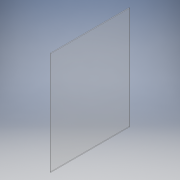
# Autodesk Inventor part: PanelThree
Saved by Autodesk Inventor 2017 (Build 210142000, 142)
## iProperties
Created: 2020-02-22
Part Number: PanelThree
Material: Polycarbonate, Clear
Document SubType Name: Modeling
Designer: S338674153
Density: 1.2 g/cm^3
Appearance: Polycarbonate - Clear
Author: S338674153
Autodesk Inventor part; units mm, degrees
ref_plane "YZ Plane" through (0, 0, 0) normal (1, 0, 0) x (0, 1, 0)
ref_plane "XZ Plane" through (0, 0, 0) normal (0, 1, 0) x (-1, 0, 0)
ref_plane "XY Plane" through (0, 0, 0) normal (0, 0, 1) x (1, 0, 0)
sketch "Sketch1" plane through (0, 0, 0) normal (0, 1, 0) x (-1, 0, 0)
  line L0 (0, 0) -> (2.54, 0)
  line L1 (2.54, 0) -> (2.54, -254)
  line L2 (2.54, -254) -> (0, -254)
  line L3 (0, -254) -> (0, 0)
  dimension "d0" = 254
  dimension "d1" = 2.54
  constraints: 8 end point, 2 parallel, 1 horizontal, 1 perpendicular
  measures "d0" distance of L0.end L1.end
  measures "d1" distance of L1.end L2.end
extrude "Extrusion1" add sketch "Sketch1" along normal blind 330.2
body "Solid1"
